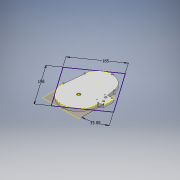
# Autodesk Inventor part: case part 1
Saved by Autodesk Inventor 2017 (Build 210142000, 142)
## iProperties
Created: 2018-04-16
Part Number: case part 1
Material: Generic
Document SubType Name: Modeling
Designer: RKL
Density: 1 g/cm^3
Appearance: Default
Mass: 277.252 g
Surface Area: 608.799 cm^2
Volume: 277.252 cm^3
Author: RKL
Autodesk Inventor part; units mm, degrees
(part 1 of 2)
ref_plane "YZ Plane" through (0, 0, 0) normal (1, 0, 0) x (0, 1, 0)
ref_plane "XZ Plane" through (0, 0, 0) normal (0, 1, 0) x (-1, 0, 0)
ref_plane "Work Plane1" through (0, 0, 0) normal (0, 0, 1) x (1, 0, 0)
sketch "Sketch1" plane through (0, 0, 0) normal (0, 0, 1) x (1, 0, 0)
  circle A0 centre (0, 0) radius 17.5 projected
  circle A1 centre (-1.6604, 79.9828) radius 17.5 projected
  circle A2 centre (0, 0) radius 6.7352 construction
  arc A3 (27.338, 58.5707) -> (27.6561, 62.122) centre (7.1943, 62.1651) ccw construction
  arc A4 (27.6561, 62.122) -> (26.5429, 62.6057) centre (0, 0) ccw construction
  arc A5 (26.5429, 62.6057) -> (24.1639, 59.95) centre (40.5363, 47.6767) ccw construction
  arc A6 (24.1639, 59.95) -> (23.09, 60.3717) centre (0, 0) ccw construction
  arc A7 (23.09, 60.3717) -> (23.1539, 63.9367) centre (2.7411, 62.5199) ccw construction
  arc A8 (23.1539, 63.9367) -> (22.009, 64.3397) centre (0, 0) ccw construction
  arc A9 (22.009, 64.3397) -> (19.8255, 61.5211) centre (37.0318, 50.447) ccw construction
  arc A10 (19.8255, 61.5211) -> (18.7243, 61.8651) centre (0, 0) ccw construction
  arc A11 (18.7243, 61.8651) -> (18.5338, 65.4255) centre (-1.726, 62.5562) ccw construction
  arc A12 (18.5338, 65.4255) -> (17.363, 65.7459) centre (0, 0) ccw construction
  arc A13 (17.363, 65.7459) -> (15.3861, 62.7787) centre (33.3386, 52.9603) ccw construction
  arc A14 (15.3861, 62.7787) -> (14.2631, 63.0433) centre (0, 0) ccw construction
  arc A15 (14.2631, 63.0433) -> (13.8191, 66.581) centre (-6.1843, 62.2737) ccw construction
  arc A16 (13.8191, 66.581) -> (12.6285, 66.8171) centre (0, 0) ccw construction
  arc A17 (12.6285, 66.8171) -> (10.8684, 63.7163) centre (29.4755, 55.2037) ccw construction
  arc A18 (10.8684, 63.7163) -> (9.7293, 63.9002) centre (0, 0) ccw construction
  arc A19 (9.7293, 63.9002) -> (9.0341, 67.3972) centre (-10.6111, 61.6738) ccw construction
  arc A20 (9.0341, 67.3972) -> (7.8297, 67.5477) centre (0, 0) ccw construction
  arc A21 (7.8297, 67.5477) -> (6.2952, 64.3293) centre (25.4622, 57.1658) ccw construction
  arc A22 (6.2952, 64.3293) -> (5.146, 64.4314) centre (0, 0) ccw construction
  arc A23 (5.146, 64.4314) -> (4.203, 67.87) centre (-14.9838, 60.7597) ccw construction
  arc A24 (4.203, 67.87) -> (2.9909, 67.9342) centre (0, 0) ccw construction
  arc A25 (2.9909, 67.9342) -> (1.6899, 64.6145) centre (21.3191, 58.8366) ccw construction
  arc A26 (1.6899, 64.6145) -> (0.5364, 64.6344) centre (0, 0) ccw construction
  arc A27 (0.5364, 64.6344) -> (-0.6495, 67.9969) centre (-19.2802, 59.536) ccw construction
  arc A28 (-0.6495, 67.9969) -> (-1.8631, 67.9745) centre (0, 0) ccw construction
  arc A29 (-1.8631, 67.9745) -> (-2.9239, 64.5704) centre (17.0675, 60.2076) ccw construction
  arc A30 (-2.9239, 64.5704) -> (-4.076, 64.508) centre (0, 0) ccw construction
  arc A31 (-4.076, 64.508) -> (-5.4987, 67.7773) centre (-23.4783, 58.0088) ccw construction
  arc A32 (-5.4987, 67.7773) -> (-6.7076, 67.6684) centre (0, 0) ccw construction
  arc A33 (-6.7076, 67.6684) -> (-7.5229, 64.1973) centre (12.7288, 61.2718) ccw construction
  arc A34 (-7.5229, 64.1973) -> (-8.6675, 64.0528) centre (0, 0) ccw construction
  arc A35 (-8.6675, 64.0528) -> (-10.3199, 67.2124) centre (-27.5568, 56.1861) ccw construction
  arc A36 (-10.3199, 67.2124) -> (-11.5179, 67.0174) centre (0, 0) ccw construction
  arc A37 (-11.5179, 67.0174) -> (-12.0835, 63.4971) centre (8.3253, 62.0238) ccw construction
  arc A38 (-12.0835, 63.4971) -> (-13.2149, 63.2713) centre (0, 0) ccw construction
  arc A39 (-13.2149, 63.2713) -> (-15.0884, 66.3049) centre (-31.4948, 54.0771) ccw construction
  arc A40 (-15.0884, 66.3049) -> (-16.2695, 66.025) centre (0, 0) ccw construction
  arc A41 (-16.2695, 66.025) -> (-16.5825, 62.4733) centre (3.8794, 62.4596) ccw construction
  arc A42 (-16.5825, 62.4733) -> (-17.695, 62.1674) centre (0, 0) ccw construction
  arc A43 (-17.695, 62.1674) -> (-19.7801, 65.0596) centre (-35.2724, 51.6925) ccw construction
  arc A44 (-19.7801, 65.0596) -> (-20.9382, 64.6961) centre (0, 0) ccw construction
  arc A45 (-20.9382, 64.6961) -> (-20.9971, 61.1311) centre (-0.5863, 62.5773) ccw construction
  arc A46 (-20.9971, 61.1311) -> (-22.0848, 60.7466) centre (0, 0) ccw construction
  arc A47 (-22.0848, 60.7466) -> (-24.371, 63.4827) centre (-38.8702, 49.0445) ccw construction
  arc A48 (-24.371, 63.4827) -> (-25.5002, 63.0376) centre (0, 0) ccw construction
  arc A49 (-25.5002, 63.0376) -> (-25.3046, 59.4775) centre (-5.049, 62.376) ccw construction
  arc A50 (-25.3046, 59.4775) -> (-26.3622, 59.0163) centre (0, 0) ccw construction
  arc A51 (-26.3622, 59.0163) -> (-28.8377, 61.5823) centre (-42.27, 46.1465) ccw construction
  arc A52 (-28.8377, 61.5823) -> (-29.9323, 61.0578) centre (0, 0) ccw construction
  arc A53 (-29.9323, 61.0578) -> (-29.4832, 57.5207) centre (-9.486, 61.8569) ccw construction
  arc A54 (-29.4832, 57.5207) -> (-30.5052, 56.9853) centre (0, 0) ccw construction
  arc A55 (-30.5052, 56.9853) -> (-33.1575, 59.3682) centre (-45.4544, 43.0135) ccw construction
  arc A56 (-33.1575, 59.3682) -> (-34.2119, 58.7669) centre (0, 0) ccw construction
  arc A57 (-34.2119, 58.7669) -> (-33.5116, 55.2708) centre (-13.8747, 61.0225) ccw construction
  arc A58 (-33.5116, 55.2708) -> (-34.4928, 54.6639) centre (0, 0) ccw construction
  arc A59 (-34.4928, 54.6639) -> (-37.3083, 56.8515) centre (-48.4071, 39.6612) ccw construction
  arc A60 (-37.3083, 56.8515) -> (-38.3171, 56.1765) centre (0, 0) ccw construction
  arc A61 (-38.3171, 56.1765) -> (-37.3692, 52.7393) centre (-18.1926, 59.8772) ccw construction
  arc A62 (-37.3692, 52.7393) -> (-38.3046, 52.0639) centre (0, 0) ccw construction
  arc A63 (-38.3046, 52.0639) -> (-41.269, 54.0451) centre (-51.1131, 36.1068) ccw construction
  arc A64 (-41.269, 54.0451) -> (-42.227, 53.2999) centre (0, 0) ccw construction
  arc A65 (-42.227, 53.2999) -> (-41.0363, 49.9391) centre (-22.4179, 58.4268) ccw construction
  arc A66 (-41.0363, 49.9391) -> (-41.9212, 49.1987) centre (0, 0) ccw construction
  arc A67 (-41.9212, 49.1987) -> (-45.0194, 50.9633) centre (-53.5587, 32.3685) ccw construction
  arc A68 (-45.0194, 50.9633) -> (-45.9218, 50.1516) centre (0, 0) ccw construction
  arc A69 (-45.9218, 50.1516) -> (-44.4944, 46.8843) centre (-26.5289, 56.6787) ccw construction
  arc A70 (-44.4944, 46.8843) -> (-45.3241, 46.0827) centre (0, 0) ccw construction
  arc A71 (-45.3241, 46.0827) -> (-48.5403, 47.6218) centre (-55.7314, 28.4651) ccw construction
  arc A72 (-48.5403, 47.6218) -> (-49.3826, 46.7478) centre (0, 0) ccw construction
  arc A73 (-49.3826, 46.7478) -> (-47.7257, 43.5907) centre (-30.5047, 54.6417) ccw construction
  arc A74 (-47.7257, 43.5907) -> (-48.4962, 42.7319) centre (0, 0) ccw construction
  arc A75 (-48.4962, 42.7319) -> (-51.814, 44.0376) centre (-57.6201, 24.4168) ccw construction
  arc A76 (-51.814, 44.0376) -> (-52.5917, 43.1058) centre (0, 0) ccw construction
  arc A77 (-52.5917, 43.1058) -> (-50.7138, 40.0749) centre (-34.3251, 52.3263) ccw construction
  arc A78 (-50.7138, 40.0749) -> (-51.4211, 39.1633) centre (0, 0) ccw construction
  arc A79 (-51.4211, 39.1633) -> (-54.8236, 40.2291) centre (-59.2152, 20.244) ccw construction
  arc A80 (-54.8236, 40.2291) -> (-55.5329, 39.2441) centre (0, 0) ccw construction
  arc A81 (-55.5329, 39.2441) -> (-53.4435, 36.3549) centre (-37.9705, 49.7443) ccw construction
  arc A82 (-53.4435, 36.3549) -> (-54.0839, 35.3952) centre (0, 0) ccw construction
  arc A83 (-54.0839, 35.3952) -> (-57.5538, 36.2155) centre (-60.5085, 15.9681) ccw construction
  arc A84 (-57.5538, 36.2155) -> (-58.191, 35.1825) centre (0, 0) ccw construction
  arc A85 (-58.191, 35.1825) -> (-55.9009, 32.4497) centre (-41.4225, 46.9088) ccw construction
  arc A86 (-55.9009, 32.4497) -> (-56.4712, 31.4467) centre (0, 0) ccw construction
  arc A87 (-56.4712, 31.4467) -> (-59.9907, 32.0174) centre (-61.4935, 11.6108) ccw construction
  arc A88 (-59.9907, 32.0174) -> (-60.5526, 30.9415) centre (0, 0) ccw construction
  arc A89 (-60.5526, 30.9415) -> (-58.0734, 28.3791) centre (-44.6634, 43.8342) ccw construction
  arc A90 (-58.0734, 28.3791) -> (-58.5707, 27.338) centre (0, 0) ccw construction
  arc A91 (-58.5707, 27.338) -> (-62.122, 27.6561) centre (-62.1651, 7.1943) ccw construction
  arc A92 (-62.122, 27.6561) -> (-62.6057, 26.5429) centre (0, 0) ccw construction
  arc A93 (-62.6057, 26.5429) -> (-59.95, 24.1639) centre (-47.6767, 40.5363) ccw construction
  arc A94 (-59.95, 24.1639) -> (-60.3717, 23.09) centre (0, 0) ccw construction
  arc A95 (-60.3717, 23.09) -> (-63.9367, 23.1539) centre (-62.5199, 2.7411) ccw construction
  arc A96 (-63.9367, 23.1539) -> (-64.3397, 22.009) centre (0, 0) ccw construction
  arc A97 (-64.3397, 22.009) -> (-61.5211, 19.8255) centre (-50.447, 37.0318) ccw construction
  arc A98 (-61.5211, 19.8255) -> (-61.8651, 18.7243) centre (0, 0) ccw construction
  arc A99 (-61.8651, 18.7243) -> (-65.4255, 18.5338) centre (-62.5562, -1.726) ccw construction
  arc A100 (-65.4255, 18.5338) -> (-65.7459, 17.363) centre (0, 0) ccw construction
  arc A101 (-65.7459, 17.363) -> (-62.7787, 15.3861) centre (-52.9603, 33.3386) ccw construction
  arc A102 (-62.7787, 15.3861) -> (-63.0433, 14.2631) centre (0, 0) ccw construction
  arc A103 (-63.0433, 14.2631) -> (-66.581, 13.8191) centre (-62.2737, -6.1843) ccw construction
  arc A104 (-66.581, 13.8191) -> (-66.8171, 12.6285) centre (0, 0) ccw construction
  arc A105 (-66.8171, 12.6285) -> (-63.7163, 10.8684) centre (-55.2037, 29.4755) ccw construction
  arc A106 (-63.7163, 10.8684) -> (-63.9002, 9.7293) centre (0, 0) ccw construction
  arc A107 (-63.9002, 9.7293) -> (-67.3972, 9.0341) centre (-61.6738, -10.6111) ccw construction
  arc A108 (-67.3972, 9.0341) -> (-67.5477, 7.8297) centre (0, 0) ccw construction
  arc A109 (-67.5477, 7.8297) -> (-64.3293, 6.2952) centre (-57.1658, 25.4622) ccw construction
  arc A110 (-64.3293, 6.2952) -> (-64.4314, 5.146) centre (0, 0) ccw construction
  arc A111 (-64.4314, 5.146) -> (-67.87, 4.203) centre (-60.7597, -14.9838) ccw construction
  arc A112 (-67.87, 4.203) -> (-67.9342, 2.9909) centre (0, 0) ccw construction
  arc A113 (-67.9342, 2.9909) -> (-64.6145, 1.6899) centre (-58.8366, 21.3191) ccw construction
  arc A114 (-64.6145, 1.6899) -> (-64.6344, 0.5364) centre (0, 0) ccw construction
  arc A115 (-64.6344, 0.5364) -> (-67.9969, -0.6495) centre (-59.536, -19.2802) ccw construction
  arc A116 (-67.9969, -0.6495) -> (-67.9745, -1.8631) centre (0, 0) ccw construction
  arc A117 (-67.9745, -1.8631) -> (-64.5704, -2.9239) centre (-60.2076, 17.0675) ccw construction
  arc A118 (-64.5704, -2.9239) -> (-64.508, -4.076) centre (0, 0) ccw construction
  arc A119 (-64.508, -4.076) -> (-67.7773, -5.4987) centre (-58.0088, -23.4783) ccw construction
  arc A120 (-67.7773, -5.4987) -> (-67.6684, -6.7076) centre (0, 0) ccw construction
  arc A121 (-67.6684, -6.7076) -> (-64.1973, -7.5229) centre (-61.2718, 12.7288) ccw construction
  arc A122 (-64.1973, -7.5229) -> (-64.0528, -8.6675) centre (0, 0) ccw construction
  arc A123 (-64.0528, -8.6675) -> (-67.2124, -10.3199) centre (-56.1861, -27.5568) ccw construction
  arc A124 (-67.2124, -10.3199) -> (-67.0174, -11.5179) centre (0, 0) ccw construction
  arc A125 (-67.0174, -11.5179) -> (-63.4971, -12.0835) centre (-62.0238, 8.3253) ccw construction
  arc A126 (-63.4971, -12.0835) -> (-63.2713, -13.2149) centre (0, 0) ccw construction
  arc A127 (-63.2713, -13.2149) -> (-66.3049, -15.0884) centre (-54.0771, -31.4948) ccw construction
  arc A128 (-66.3049, -15.0884) -> (-66.025, -16.2695) centre (0, 0) ccw construction
  arc A129 (-66.025, -16.2695) -> (-62.4733, -16.5825) centre (-62.4596, 3.8794) ccw construction
  arc A130 (-62.4733, -16.5825) -> (-62.1674, -17.695) centre (0, 0) ccw construction
  arc A131 (-62.1674, -17.695) -> (-65.0596, -19.7801) centre (-51.6925, -35.2724) ccw construction
  arc A132 (-65.0596, -19.7801) -> (-64.6961, -20.9382) centre (0, 0) ccw construction
  arc A133 (-64.6961, -20.9382) -> (-61.1311, -20.9971) centre (-62.5773, -0.5863) ccw construction
  arc A134 (-61.1311, -20.9971) -> (-60.7466, -22.0848) centre (0, 0) ccw construction
  arc A135 (-60.7466, -22.0848) -> (-63.4827, -24.371) centre (-49.0445, -38.8702) ccw construction
  arc A136 (-63.4827, -24.371) -> (-63.0376, -25.5002) centre (0, 0) ccw construction
  arc A137 (-63.0376, -25.5002) -> (-59.4775, -25.3046) centre (-62.376, -5.049) ccw construction
  arc A138 (-59.4775, -25.3046) -> (-59.0163, -26.3622) centre (0, 0) ccw construction
  arc A139 (-59.0163, -26.3622) -> (-61.5823, -28.8377) centre (-46.1465, -42.27) ccw construction
  arc A140 (-61.5823, -28.8377) -> (-61.0578, -29.9323) centre (0, 0) ccw construction
  arc A141 (-61.0578, -29.9323) -> (-57.5207, -29.4832) centre (-61.8569, -9.486) ccw construction
  arc A142 (-57.5207, -29.4832) -> (-56.9853, -30.5052) centre (0, 0) ccw construction
  arc A143 (-56.9853, -30.5052) -> (-59.3682, -33.1575) centre (-43.0135, -45.4544) ccw construction
  arc A144 (-59.3682, -33.1575) -> (-58.7669, -34.2119) centre (0, 0) ccw construction
  arc A145 (-58.7669, -34.2119) -> (-55.2708, -33.5116) centre (-61.0225, -13.8747) ccw construction
  arc A146 (-55.2708, -33.5116) -> (-54.6639, -34.4928) centre (0, 0) ccw construction
  arc A147 (-54.6639, -34.4928) -> (-56.8515, -37.3083) centre (-39.6612, -48.4071) ccw construction
  arc A148 (-56.8515, -37.3083) -> (-56.1765, -38.3171) centre (0, 0) ccw construction
  arc A149 (-56.1765, -38.3171) -> (-52.7393, -37.3692) centre (-59.8772, -18.1926) ccw construction
  arc A150 (-52.7393, -37.3692) -> (-52.0639, -38.3046) centre (0, 0) ccw construction
  arc A151 (-52.0639, -38.3046) -> (-54.0451, -41.269) centre (-36.1068, -51.1131) ccw construction
  arc A152 (-54.0451, -41.269) -> (-53.2999, -42.227) centre (0, 0) ccw construction
  arc A153 (-53.2999, -42.227) -> (-49.9391, -41.0363) centre (-58.4268, -22.4179) ccw construction
  arc A154 (-49.9391, -41.0363) -> (-49.1987, -41.9212) centre (0, 0) ccw construction
  arc A155 (-49.1987, -41.9212) -> (-50.9633, -45.0194) centre (-32.3685, -53.5587) ccw construction
  arc A156 (-50.9633, -45.0194) -> (-50.1516, -45.9218) centre (0, 0) ccw construction
  arc A157 (-50.1516, -45.9218) -> (-46.8843, -44.4944) centre (-56.6787, -26.5289) ccw construction
  arc A158 (-46.8843, -44.4944) -> (-46.0827, -45.3241) centre (0, 0) ccw construction
  arc A159 (-46.0827, -45.3241) -> (-47.6218, -48.5403) centre (-28.4651, -55.7314) ccw construction
  arc A160 (-47.6218, -48.5403) -> (-46.7478, -49.3826) centre (0, 0) ccw construction
  arc A161 (-46.7478, -49.3826) -> (-43.5907, -47.7257) centre (-54.6417, -30.5047) ccw construction
  arc A162 (-43.5907, -47.7257) -> (-42.7319, -48.4962) centre (0, 0) ccw construction
  arc A163 (-42.7319, -48.4962) -> (-44.0376, -51.814) centre (-24.4168, -57.6201) ccw construction
  arc A164 (-44.0376, -51.814) -> (-43.1058, -52.5917) centre (0, 0) ccw construction
  arc A165 (-43.1058, -52.5917) -> (-40.0749, -50.7138) centre (-52.3263, -34.3251) ccw construction
  arc A166 (-40.0749, -50.7138) -> (-39.1633, -51.4211) centre (0, 0) ccw construction
  arc A167 (-39.1633, -51.4211) -> (-40.2291, -54.8236) centre (-20.244, -59.2152) ccw construction
  arc A168 (-40.2291, -54.8236) -> (-39.2441, -55.5329) centre (0, 0) ccw construction
  arc A169 (-39.2441, -55.5329) -> (-36.3549, -53.4435) centre (-49.7443, -37.9705) ccw construction
  arc A170 (-36.3549, -53.4435) -> (-35.3952, -54.0839) centre (0, 0) ccw construction
  arc A171 (-35.3952, -54.0839) -> (-36.2155, -57.5538) centre (-15.9681, -60.5085) ccw construction
  arc A172 (-36.2155, -57.5538) -> (-35.1825, -58.191) centre (0, 0) ccw construction
  arc A173 (-35.1825, -58.191) -> (-32.4497, -55.9009) centre (-46.9088, -41.4225) ccw construction
  arc A174 (-32.4497, -55.9009) -> (-31.4467, -56.4712) centre (0, 0) ccw construction
  arc A175 (-31.4467, -56.4712) -> (-32.0174, -59.9907) centre (-11.6108, -61.4935) ccw construction
  arc A176 (-32.0174, -59.9907) -> (-30.9415, -60.5526) centre (0, 0) ccw construction
  arc A177 (-30.9415, -60.5526) -> (-28.3791, -58.0734) centre (-43.8342, -44.6634) ccw construction
  arc A178 (-28.3791, -58.0734) -> (-27.338, -58.5707) centre (0, 0) ccw construction
  arc A179 (-27.338, -58.5707) -> (-27.6561, -62.122) centre (-7.1943, -62.1651) ccw construction
  arc A180 (-27.6561, -62.122) -> (-26.5429, -62.6057) centre (0, 0) ccw construction
  arc A181 (-26.5429, -62.6057) -> (-24.1639, -59.95) centre (-40.5363, -47.6767) ccw construction
  arc A182 (-24.1639, -59.95) -> (-23.09, -60.3717) centre (0, 0) ccw construction
  arc A183 (-23.09, -60.3717) -> (-23.1539, -63.9367) centre (-2.7411, -62.5199) ccw construction
  arc A184 (-23.1539, -63.9367) -> (-22.009, -64.3397) centre (0, 0) ccw construction
  arc A185 (-22.009, -64.3397) -> (-19.8255, -61.5211) centre (-37.0318, -50.447) ccw construction
  arc A186 (-19.8255, -61.5211) -> (-18.7243, -61.8651) centre (0, 0) ccw construction
  arc A187 (-18.7243, -61.8651) -> (-18.5338, -65.4255) centre (1.726, -62.5562) ccw construction
  arc A188 (-18.5338, -65.4255) -> (-17.363, -65.7459) centre (0, 0) ccw construction
  arc A189 (-17.363, -65.7459) -> (-15.3861, -62.7787) centre (-33.3386, -52.9603) ccw construction
  arc A190 (-15.3861, -62.7787) -> (-14.2631, -63.0433) centre (0, 0) ccw construction
  arc A191 (-14.2631, -63.0433) -> (-13.8191, -66.581) centre (6.1843, -62.2737) ccw construction
  arc A192 (-13.8191, -66.581) -> (-12.6285, -66.8171) centre (0, 0) ccw construction
  arc A193 (-12.6285, -66.8171) -> (-10.8684, -63.7163) centre (-29.4755, -55.2037) ccw construction
  arc A194 (-10.8684, -63.7163) -> (-9.7293, -63.9002) centre (0, 0) ccw construction
  arc A195 (-9.7293, -63.9002) -> (-9.0341, -67.3972) centre (10.6111, -61.6738) ccw construction
  arc A196 (-9.0341, -67.3972) -> (-7.8297, -67.5477) centre (0, 0) ccw construction
  arc A197 (-7.8297, -67.5477) -> (-6.2952, -64.3293) centre (-25.4622, -57.1658) ccw construction
  arc A198 (-6.2952, -64.3293) -> (-5.146, -64.4314) centre (0, 0) ccw construction
  arc A199 (-5.146, -64.4314) -> (-4.203, -67.87) centre (14.9838, -60.7597) ccw construction
  arc A200 (-4.203, -67.87) -> (-2.9909, -67.9342) centre (0, 0) ccw construction
  arc A201 (-2.9909, -67.9342) -> (-1.6899, -64.6145) centre (-21.3191, -58.8366) ccw construction
  arc A202 (-1.6899, -64.6145) -> (-0.5364, -64.6344) centre (0, 0) ccw construction
  arc A203 (-0.5364, -64.6344) -> (0.6495, -67.9969) centre (19.2802, -59.536) ccw construction
  arc A204 (0.6495, -67.9969) -> (1.8631, -67.9745) centre (0, 0) ccw construction
  arc A205 (1.8631, -67.9745) -> (2.9239, -64.5704) centre (-17.0675, -60.2076) ccw construction
  arc A206 (2.9239, -64.5704) -> (4.076, -64.508) centre (0, 0) ccw construction
  arc A207 (4.076, -64.508) -> (5.4987, -67.7773) centre (23.4783, -58.0088) ccw construction
  arc A208 (5.4987, -67.7773) -> (6.7076, -67.6684) centre (0, 0) ccw construction
  arc A209 (6.7076, -67.6684) -> (7.5229, -64.1973) centre (-12.7288, -61.2718) ccw construction
  arc A210 (7.5229, -64.1973) -> (8.6675, -64.0528) centre (0, 0) ccw construction
  arc A211 (8.6675, -64.0528) -> (10.3199, -67.2124) centre (27.5568, -56.1861) ccw construction
  arc A212 (10.3199, -67.2124) -> (11.5179, -67.0174) centre (0, 0) ccw construction
  arc A213 (11.5179, -67.0174) -> (12.0835, -63.4971) centre (-8.3253, -62.0238) ccw construction
  arc A214 (12.0835, -63.4971) -> (13.2149, -63.2713) centre (0, 0) ccw construction
  arc A215 (13.2149, -63.2713) -> (15.0884, -66.3049) centre (31.4948, -54.0771) ccw construction
  arc A216 (15.0884, -66.3049) -> (16.2695, -66.025) centre (0, 0) ccw construction
  arc A217 (16.2695, -66.025) -> (16.5825, -62.4733) centre (-3.8794, -62.4596) ccw construction
  arc A218 (16.5825, -62.4733) -> (17.695, -62.1674) centre (0, 0) ccw construction
  arc A219 (17.695, -62.1674) -> (19.7801, -65.0596) centre (35.2724, -51.6925) ccw construction
  arc A220 (19.7801, -65.0596) -> (20.9382, -64.6961) centre (0, 0) ccw construction
  arc A221 (20.9382, -64.6961) -> (20.9971, -61.1311) centre (0.5863, -62.5773) ccw construction
  arc A222 (20.9971, -61.1311) -> (22.0848, -60.7466) centre (0, 0) ccw construction
  arc A223 (22.0848, -60.7466) -> (24.371, -63.4827) centre (38.8702, -49.0445) ccw construction
  arc A224 (24.371, -63.4827) -> (25.5002, -63.0376) centre (0, 0) ccw construction
  arc A225 (25.5002, -63.0376) -> (25.3046, -59.4775) centre (5.049, -62.376) ccw construction
  arc A226 (25.3046, -59.4775) -> (26.3622, -59.0163) centre (0, 0) ccw construction
  arc A227 (26.3622, -59.0163) -> (28.8377, -61.5823) centre (42.27, -46.1465) ccw construction
  arc A228 (28.8377, -61.5823) -> (29.9323, -61.0578) centre (0, 0) ccw construction
  arc A229 (29.9323, -61.0578) -> (29.4832, -57.5207) centre (9.486, -61.8569) ccw construction
  arc A230 (29.4832, -57.5207) -> (30.5052, -56.9853) centre (0, 0) ccw construction
  arc A231 (30.5052, -56.9853) -> (33.1575, -59.3682) centre (45.4544, -43.0135) ccw construction
  arc A232 (33.1575, -59.3682) -> (34.2119, -58.7669) centre (0, 0) ccw construction
  arc A233 (34.2119, -58.7669) -> (33.5116, -55.2708) centre (13.8747, -61.0225) ccw construction
  arc A234 (33.5116, -55.2708) -> (34.4928, -54.6639) centre (0, 0) ccw construction
  arc A235 (34.4928, -54.6639) -> (37.3083, -56.8515) centre (48.4071, -39.6612) ccw construction
  arc A236 (37.3083, -56.8515) -> (38.3171, -56.1765) centre (0, 0) ccw construction
  arc A237 (38.3171, -56.1765) -> (37.3692, -52.7393) centre (18.1926, -59.8772) ccw construction
  arc A238 (37.3692, -52.7393) -> (38.3046, -52.0639) centre (0, 0) ccw construction
  arc A239 (38.3046, -52.0639) -> (41.269, -54.0451) centre (51.1131, -36.1068) ccw construction
  arc A240 (41.269, -54.0451) -> (42.227, -53.2999) centre (0, 0) ccw construction
  arc A241 (42.227, -53.2999) -> (41.0363, -49.9391) centre (22.4179, -58.4268) ccw construction
  arc A242 (41.0363, -49.9391) -> (41.9212, -49.1987) centre (0, 0) ccw construction
  arc A243 (41.9212, -49.1987) -> (45.0194, -50.9633) centre (53.5587, -32.3685) ccw construction
  arc A244 (45.0194, -50.9633) -> (45.9218, -50.1516) centre (0, 0) ccw construction
  arc A245 (45.9218, -50.1516) -> (44.4944, -46.8843) centre (26.5289, -56.6787) ccw construction
  arc A246 (44.4944, -46.8843) -> (45.3241, -46.0827) centre (0, 0) ccw construction
  arc A247 (45.3241, -46.0827) -> (48.5403, -47.6218) centre (55.7314, -28.4651) ccw construction
  arc A248 (48.5403, -47.6218) -> (49.3826, -46.7478) centre (0, 0) ccw construction
  arc A249 (49.3826, -46.7478) -> (47.7257, -43.5907) centre (30.5047, -54.6417) ccw construction
  arc A250 (47.7257, -43.5907) -> (48.4962, -42.7319) centre (0, 0) ccw construction
  arc A251 (48.4962, -42.7319) -> (51.814, -44.0376) centre (57.6201, -24.4168) ccw construction
  arc A252 (51.814, -44.0376) -> (52.5917, -43.1058) centre (0, 0) ccw construction
  arc A253 (52.5917, -43.1058) -> (50.7138, -40.0749) centre (34.3251, -52.3263) ccw construction
  arc A254 (50.7138, -40.0749) -> (51.4211, -39.1633) centre (0, 0) ccw construction
  arc A255 (51.4211, -39.1633) -> (54.8236, -40.2291) centre (59.2152, -20.244) ccw construction
  arc A256 (54.8236, -40.2291) -> (55.5329, -39.2441) centre (0, 0) ccw construction
  arc A257 (55.5329, -39.2441) -> (53.4435, -36.3549) centre (37.9705, -49.7443) ccw construction
  arc A258 (53.4435, -36.3549) -> (54.0839, -35.3952) centre (0, 0) ccw construction
  arc A259 (54.0839, -35.3952) -> (57.5538, -36.2155) centre (60.5085, -15.9681) ccw construction
  arc A260 (57.5538, -36.2155) -> (58.191, -35.1825) centre (0, 0) ccw construction
  arc A261 (58.191, -35.1825) -> (55.9009, -32.4497) centre (41.4225, -46.9088) ccw construction
  arc A262 (55.9009, -32.4497) -> (56.4712, -31.4467) centre (0, 0) ccw construction
  arc A263 (56.4712, -31.4467) -> (59.9907, -32.0174) centre (61.4935, -11.6108) ccw construction
  arc A264 (59.9907, -32.0174) -> (60.5526, -30.9415) centre (0, 0) ccw construction
  arc A265 (60.5526, -30.9415) -> (58.0734, -28.3791) centre (44.6634, -43.8342) ccw construction
  arc A266 (58.0734, -28.3791) -> (58.5707, -27.338) centre (0, 0) ccw construction
  arc A267 (58.5707, -27.338) -> (62.122, -27.6561) centre (62.1651, -7.1943) ccw construction
  arc A268 (62.122, -27.6561) -> (62.6057, -26.5429) centre (0, 0) ccw construction
  arc A269 (62.6057, -26.5429) -> (59.95, -24.1639) centre (47.6767, -40.5363) ccw construction
  arc A270 (59.95, -24.1639) -> (60.3717, -23.09) centre (0, 0) ccw construction
  arc A271 (60.3717, -23.09) -> (63.9367, -23.1539) centre (62.5199, -2.7411) ccw construction
  arc A272 (63.9367, -23.1539) -> (64.3397, -22.009) centre (0, 0) ccw construction
  arc A273 (64.3397, -22.009) -> (61.5211, -19.8255) centre (50.447, -37.0318) ccw construction
  arc A274 (61.5211, -19.8255) -> (61.8651, -18.7243) centre (0, 0) ccw construction
  arc A275 (61.8651, -18.7243) -> (65.4255, -18.5338) centre (62.5562, 1.726) ccw construction
  arc A276 (65.4255, -18.5338) -> (65.7459, -17.363) centre (0, 0) ccw construction
  arc A277 (65.7459, -17.363) -> (62.7787, -15.3861) centre (52.9603, -33.3386) ccw construction
  arc A278 (62.7787, -15.3861) -> (63.0433, -14.2631) centre (0, 0) ccw construction
  arc A279 (63.0433, -14.2631) -> (66.581, -13.8191) centre (62.2737, 6.1843) ccw construction
  arc A280 (66.581, -13.8191) -> (66.8171, -12.6285) centre (0, 0) ccw construction
  arc A281 (66.8171, -12.6285) -> (63.7163, -10.8684) centre (55.2037, -29.4755) ccw construction
  arc A282 (63.7163, -10.8684) -> (63.9002, -9.7293) centre (0, 0) ccw construction
  arc A283 (63.9002, -9.7293) -> (67.3972, -9.0341) centre (61.6738, 10.6111) ccw construction
  arc A284 (67.3972, -9.0341) -> (67.5477, -7.8297) centre (0, 0) ccw construction
  arc A285 (67.5477, -7.8297) -> (64.3293, -6.2952) centre (57.1658, -25.4622) ccw construction
  arc A286 (64.3293, -6.2952) -> (64.4314, -5.146) centre (0, 0) ccw construction
  arc A287 (64.4314, -5.146) -> (67.87, -4.203) centre (60.7597, 14.9838) ccw construction
  arc A288 (67.87, -4.203) -> (67.9342, -2.9909) centre (0, 0) ccw construction
  arc A289 (67.9342, -2.9909) -> (64.6145, -1.6899) centre (58.8366, -21.3191) ccw construction
  arc A290 (64.6145, -1.6899) -> (64.6344, -0.5364) centre (0, 0) ccw construction
  arc A291 (64.6344, -0.5364) -> (67.9969, 0.6495) centre (59.536, 19.2802) ccw construction
  arc A292 (67.9969, 0.6495) -> (67.9745, 1.8631) centre (0, 0) ccw construction
  arc A293 (67.9745, 1.8631) -> (64.5704, 2.9239) centre (60.2076, -17.0675) ccw construction
  arc A294 (64.5704, 2.9239) -> (64.508, 4.076) centre (0, 0) ccw construction
  arc A295 (64.508, 4.076) -> (67.7773, 5.4987) centre (58.0088, 23.4783) ccw construction
  arc A296 (67.7773, 5.4987) -> (67.6684, 6.7076) centre (0, 0) ccw construction
  arc A297 (67.6684, 6.7076) -> (64.1973, 7.5229) centre (61.2718, -12.7288) ccw construction
  arc A298 (64.1973, 7.5229) -> (64.0528, 8.6675) centre (0, 0) ccw construction
  arc A299 (64.0528, 8.6675) -> (67.2124, 10.3199) centre (56.1861, 27.5568) ccw construction
  arc A300 (67.2124, 10.3199) -> (67.0174, 11.5179) centre (0, 0) ccw construction
  arc A301 (67.0174, 11.5179) -> (63.4971, 12.0835) centre (62.0238, -8.3253) ccw construction
  arc A302 (63.4971, 12.0835) -> (63.2713, 13.2149) centre (0, 0) ccw construction
  arc A303 (63.2713, 13.2149) -> (66.3049, 15.0884) centre (54.0771, 31.4948) ccw construction
  arc A304 (66.3049, 15.0884) -> (66.025, 16.2695) centre (0, 0) ccw construction
  arc A305 (66.025, 16.2695) -> (62.4733, 16.5825) centre (62.4596, -3.8794) ccw construction
  arc A306 (62.4733, 16.5825) -> (62.1674, 17.695) centre (0, 0) ccw construction
  arc A307 (62.1674, 17.695) -> (65.0596, 19.7801) centre (51.6925, 35.2724) ccw construction
  arc A308 (65.0596, 19.7801) -> (64.6961, 20.9382) centre (0, 0) ccw construction
  arc A309 (64.6961, 20.9382) -> (61.1311, 20.9971) centre (62.5773, 0.5863) ccw construction
  arc A310 (61.1311, 20.9971) -> (60.7466, 22.0848) centre (0, 0) ccw construction
  arc A311 (60.7466, 22.0848) -> (63.4827, 24.371) centre (49.0445, 38.8702) ccw construction
  arc A312 (63.4827, 24.371) -> (63.0376, 25.5002) centre (0, 0) ccw construction
  arc A313 (63.0376, 25.5002) -> (59.4775, 25.3046) centre (62.376, 5.049) ccw construction
  arc A314 (59.4775, 25.3046) -> (59.0163, 26.3622) centre (0, 0) ccw construction
  arc A315 (59.0163, 26.3622) -> (61.5823, 28.8377) centre (46.1465, 42.27) ccw construction
  arc A316 (61.5823, 28.8377) -> (61.0578, 29.9323) centre (0, 0) ccw construction
  arc A317 (61.0578, 29.9323) -> (57.5207, 29.4832) centre (61.8569, 9.486) ccw construction
  arc A318 (57.5207, 29.4832) -> (56.9853, 30.5052) centre (0, 0) ccw construction
  arc A319 (56.9853, 30.5052) -> (59.3682, 33.1575) centre (43.0135, 45.4544) ccw construction
  arc A320 (59.3682, 33.1575) -> (58.7669, 34.2119) centre (0, 0) ccw construction
  arc A321 (58.7669, 34.2119) -> (55.2708, 33.5116) centre (61.0225, 13.8747) ccw construction
  arc A322 (55.2708, 33.5116) -> (54.6639, 34.4928) centre (0, 0) ccw construction
  arc A323 (54.6639, 34.4928) -> (56.8515, 37.3083) centre (39.6612, 48.4071) ccw construction
  arc A324 (56.8515, 37.3083) -> (56.1765, 38.3171) centre (0, 0) ccw construction
  arc A325 (56.1765, 38.3171) -> (52.7393, 37.3692) centre (59.8772, 18.1926) ccw construction
  arc A326 (52.7393, 37.3692) -> (52.0639, 38.3046) centre (0, 0) ccw construction
  arc A327 (52.0639, 38.3046) -> (54.0451, 41.269) centre (36.1068, 51.1131) ccw construction
  arc A328 (54.0451, 41.269) -> (53.2999, 42.227) centre (0, 0) ccw construction
  arc A329 (53.2999, 42.227) -> (49.9391, 41.0363) centre (58.4268, 22.4179) ccw construction
  arc A330 (49.9391, 41.0363) -> (49.1987, 41.9212) centre (0, 0) ccw construction
  arc A331 (49.1987, 41.9212) -> (50.9633, 45.0194) centre (32.3685, 53.5587) ccw construction
  arc A332 (50.9633, 45.0194) -> (50.1516, 45.9218) centre (0, 0) ccw construction
  arc A333 (50.1516, 45.9218) -> (46.8843, 44.4944) centre (56.6787, 26.5289) ccw construction
  arc A334 (46.8843, 44.4944) -> (46.0827, 45.3241) centre (0, 0) ccw construction
  arc A335 (46.0827, 45.3241) -> (47.6218, 48.5403) centre (28.4651, 55.7314) ccw construction
  arc A336 (47.6218, 48.5403) -> (46.7478, 49.3826) centre (0, 0) ccw construction
  arc A337 (46.7478, 49.3826) -> (43.5907, 47.7257) centre (54.6417, 30.5047) ccw construction
  arc A338 (43.5907, 47.7257) -> (42.7319, 48.4962) centre (0, 0) ccw construction
  arc A339 (42.7319, 48.4962) -> (44.0376, 51.814) centre (24.4168, 57.6201) ccw construction
  arc A340 (44.0376, 51.814) -> (43.1058, 52.5917) centre (0, 0) ccw construction
  arc A341 (43.1058, 52.5917) -> (40.0749, 50.7138) centre (52.3263, 34.3251) ccw construction
  arc A342 (40.0749, 50.7138) -> (39.1633, 51.4211) centre (0, 0) ccw construction
  arc A343 (39.1633, 51.4211) -> (40.2291, 54.8236) centre (20.244, 59.2152) ccw construction
  arc A344 (40.2291, 54.8236) -> (39.2441, 55.5329) centre (0, 0) ccw construction
  arc A345 (39.2441, 55.5329) -> (36.3549, 53.4435) centre (49.7443, 37.9705) ccw construction
  arc A346 (36.3549, 53.4435) -> (35.3952, 54.0839) centre (0, 0) ccw construction
  arc A347 (35.3952, 54.0839) -> (36.2155, 57.5538) centre (15.9681, 60.5085) ccw construction
  arc A348 (36.2155, 57.5538) -> (35.1825, 58.191) centre (0, 0) ccw construction
  arc A349 (35.1825, 58.191) -> (32.4497, 55.9009) centre (46.9088, 41.4225) ccw construction
  arc A350 (32.4497, 55.9009) -> (31.4467, 56.4712) centre (0, 0) ccw construction
  arc A351 (31.4467, 56.4712) -> (32.0174, 59.9907) centre (11.6108, 61.4935) ccw construction
  arc A352 (32.0174, 59.9907) -> (30.9415, 60.5526) centre (0, 0) ccw construction
  arc A353 (30.9415, 60.5526) -> (28.3791, 58.0734) centre (43.8342, 44.6634) ccw construction
  arc A354 (28.3791, 58.0734) -> (27.338, 58.5707) centre (0, 0) ccw construction
  line L0 (-2.3049, 86.687) -> (5.0439, 80.6273) construction
  line L1 (5.0439, 80.6273) -> (-1.0158, 73.2785) construction
  line L2 (-1.0158, 73.2785) -> (-8.3646, 79.3382) construction
  line L3 (-8.3646, 79.3382) -> (-2.3049, 86.687) construction
  arc A355 (37.216, 46.5883) -> (38.5292, 48.1808) centre (-1.6604, 79.9828) ccw construction
  arc A356 (32.9073, 42.1458) -> (30.4447, 47.5651) centre (6.6438, 33.4802) ccw construction
  arc A357 (30.4447, 47.5651) -> (31.724, 48.8841) centre (-1.6604, 79.9828) ccw construction
  arc A358 (31.724, 48.8841) -> (37.216, 46.5883) centre (45.0744, 73.1046) ccw construction
  arc A359 (38.5292, 48.1808) -> (35.2291, 53.1349) centre (13.9958, 35.4145) ccw construction
  arc A360 (35.2291, 53.1349) -> (36.2802, 54.642) centre (-1.6604, 79.9828) ccw construction
  arc A361 (36.2802, 54.642) -> (42.0694, 53.257) centre (45.5725, 80.6905) ccw construction
  arc A362 (42.0694, 53.257) -> (43.1101, 55.0395) centre (-1.6604, 79.9828) ccw construction
  arc A363 (43.1101, 55.0395) -> (39.0581, 59.4) centre (20.9423, 38.503) ccw construction
  arc A364 (39.0581, 59.4) -> (39.8538, 61.0563) centre (-1.6604, 79.9828) ccw construction
  arc A365 (39.8538, 61.0563) -> (45.7903, 60.6178) centre (44.8473, 88.258) ccw construction
  arc A366 (45.7903, 60.6178) -> (46.5315, 62.5442) centre (-1.6604, 79.9828) ccw construction
  arc A367 (46.5315, 62.5442) -> (41.8325, 66.1983) centre (27.3034, 42.6659) ccw construction
  arc A368 (41.8325, 66.1983) -> (42.3523, 67.9607) centre (-1.6604, 79.9828) ccw construction
  arc A369 (42.3523, 67.9607) -> (48.2821, 68.4802) centre (42.9176, 95.6112) ccw construction
  arc A370 (48.2821, 68.4802) -> (48.7048, 70.5005) centre (-1.6604, 79.9828) ccw construction
  arc A371 (48.7048, 70.5005) -> (43.4805, 73.3535) centre (32.9144, 47.7953) ccw construction
  arc A372 (43.4805, 73.3535) -> (43.7108, 75.1765) centre (-1.6604, 79.9828) ccw construction
  arc A373 (43.7108, 75.1765) -> (49.4805, 76.6405) centre (39.8334, 102.5596) ccw construction
  arc A374 (49.4805, 76.6405) -> (49.5736, 78.7025) centre (-1.6604, 79.9828) ccw construction
  arc A375 (49.5736, 78.7025) -> (43.9593, 80.6805) centre (37.6299, 53.7583) ccw construction
  arc A376 (43.9593, 80.6805) -> (43.8942, 82.5168) centre (-1.6604, 79.9828) ccw construction
  arc A377 (43.8942, 82.5168) -> (49.3544, 84.8874) centre (35.6745, 108.9233) ccw construction
  arc A378 (49.3544, 84.8874) -> (49.1155, 86.9376) centre (-1.6604, 79.9828) ccw construction
  arc A379 (49.1155, 86.9376) -> (43.2566, 87.9893) centre (41.3278, 60.4005) ccw construction
  arc A380 (43.2566, 87.9893) -> (42.8978, 89.7915) centre (-1.6604, 79.9828) ccw construction
  arc A381 (42.8978, 89.7915) -> (47.907, 93.0072) centre (30.5486, 114.5375) ccw construction
  arc A382 (47.907, 93.0072) -> (47.3424, 94.9925) centre (-1.6604, 79.9828) ccw construction
  arc A383 (47.3424, 94.9925) -> (41.3906, 95.0908) centre (43.9123, 67.5498) ccw construction
  arc A384 (41.3906, 95.0908) -> (40.7474, 96.8121) centre (-1.6604, 79.9828) ccw construction
  arc A385 (40.7474, 96.8121) -> (45.1759, 100.7897) centre (24.5886, 119.2567) ccw construction
  arc A386 (45.1759, 100.7897) -> (44.3001, 102.6587) centre (-1.6604, 79.9828) ccw construction
  arc A387 (44.3001, 102.6587) -> (38.4096, 101.8011) centre (45.3165, 75.0212) ccw construction
  arc A388 (38.4096, 101.8011) -> (37.4986, 103.3968) centre (-1.6604, 79.9828) ccw construction
  arc A389 (37.4986, 103.3968) -> (41.2317, 108.0333) centre (17.9487, 122.9587) ccw construction
  arc A390 (41.2317, 108.0333) -> (40.0674, 109.7377) centre (-1.6604, 79.9828) ccw construction
  arc A391 (40.0674, 109.7377) -> (34.3908, 107.9462) centre (45.5041, 82.6211) ccw construction
  arc A392 (34.3908, 107.9462) -> (33.2356, 109.3752) centre (-1.6604, 79.9828) ccw construction
  arc A393 (33.2356, 109.3752) -> (36.1766, 114.5504) centre (10.8009, 125.5477) ccw construction
  arc A394 (36.1766, 114.5504) -> (34.754, 116.046) centre (-1.6604, 79.9828) ccw construction
  arc A395 (34.754, 116.046) -> (29.4383, 113.3671) centre (44.4701, 90.1526) ccw construction
  arc A396 (29.4383, 113.3671) -> (28.0688, 114.5922) centre (-1.6604, 79.9828) ccw construction
  arc A397 (28.0688, 114.5922) -> (30.1416, 120.1723) centre (3.3304, 126.9566) ccw construction
  arc A398 (30.1416, 120.1723) -> (28.4975, 121.4202) centre (-1.6604, 79.9828) ccw construction
  arc A399 (28.4975, 121.4202) -> (23.6804, 117.9234) centre (42.2414, 97.4208) ccw construction
  arc A400 (23.6804, 117.9234) -> (22.1321, 118.913) centre (-1.6604, 79.9828) ccw construction
  arc A401 (22.1321, 118.913) -> (23.2829, 124.7532) centre (-4.2694, 127.1489) ccw construction
  arc A402 (23.2829, 124.7532) -> (21.46, 125.7213) centre (-1.6604, 79.9828) ccw construction
  arc A403 (21.46, 125.7213) -> (17.2661, 121.497) centre (38.8756, 104.2373) ccw construction
  arc A404 (17.2661, 121.497) -> (15.5791, 122.2254) centre (-1.6604, 79.9828) ccw construction
  arc A405 (15.5791, 122.2254) -> (15.7782, 128.1747) centre (-11.8015, 126.1196) ccw construction
  arc A406 (15.7782, 128.1747) -> (13.8236, 128.8378) centre (-1.6604, 79.9828) ccw construction
  arc A407 (13.8236, 128.8378) -> (10.3617, 123.9954) centre (34.46, 110.4256) ccw construction
  arc A408 (10.3617, 123.9954) -> (8.5797, 124.4438) centre (-1.6604, 79.9828) ccw construction
  arc A409 (8.5797, 124.4438) -> (7.8219, 130.3479) centre (-19.0711, 123.8953) ccw construction
  arc A410 (7.8219, 130.3479) -> (5.7862, 130.6889) centre (-1.6604, 79.9828) ccw construction
  arc A411 (5.7862, 130.6889) -> (3.1459, 125.3539) centre (29.1088, 115.8255) ccw construction
  arc A412 (3.1459, 125.3539) -> (1.3151, 125.5106) centre (-1.6604, 79.9828) ccw construction
  arc A413 (1.3151, 125.5106) -> (-0.3801, 131.2168) centre (-25.8897, 120.5338) ccw construction
  arc A414 (-0.3801, 131.2168) -> (-2.4441, 131.2268) centre (-1.6604, 79.9828) ccw construction
  arc A415 (-2.4441, 131.2268) -> (-4.1944, 125.5373) centre (22.9608, 120.2971) ccw construction
  arc A416 (-4.1944, 125.5373) -> (-6.0267, 125.3984) centre (-1.6604, 79.9828) ccw construction
  arc A417 (-6.0267, 125.3984) -> (-8.6152, 130.7587) centre (-32.0808, 116.122) ccw construction
  arc A418 (-8.6152, 130.7587) -> (-10.6541, 130.4375) centre (-1.6604, 79.9828) ccw construction
  arc A419 (-10.6541, 130.4375) -> (-11.4691, 124.5409) centre (16.1751, 123.7245) ccw construction
  arc A420 (-11.4691, 124.5409) -> (-13.2553, 124.1098) centre (-1.6604, 79.9828) ccw construction
  arc A421 (-13.2553, 124.1098) -> (-16.6701, 128.9855) centre (-37.484, 110.7743) ccw construction
  arc A422 (-16.6701, 128.9855) -> (-18.6311, 128.3414) centre (-1.6604, 79.9828) ccw construction
  arc A423 (-18.6311, 128.3414) -> (-18.4897, 122.3905) centre (8.9275, 126.0191) ccw construction
  arc A424 (-18.4897, 122.3905) -> (-20.1836, 121.6784) centre (-1.6604, 79.9828) ccw construction
  arc A425 (-20.1836, 121.6784) -> (-24.3363, 125.9432) centre (-41.9594, 104.629) ccw construction
  arc A426 (-24.3363, 125.9432) -> (-26.1686, 124.9929) centre (-1.6604, 79.9828) ccw construction
  arc A427 (-26.1686, 124.9929) -> (-25.0744, 119.1417) centre (1.4056, 127.1214) ccw construction
  arc A428 (-25.0744, 119.1417) -> (-26.6322, 118.1672) centre (-1.6604, 79.9828) ccw construction
  arc A429 (-26.6322, 118.1672) -> (-31.4153, 121.7106) centre (-45.391, 97.8454) ccw construction
  arc A430 (-31.4153, 121.7106) -> (-33.0713, 120.4786) centre (-1.6604, 79.9828) ccw construction
  arc A431 (-33.0713, 120.4786) -> (-31.0528, 114.8787) centre (-6.1957, 127.0027) ccw construction
  arc A432 (-31.0528, 114.8787) -> (-32.434, 113.6669) centre (-1.6604, 79.9828) ccw construction
  arc A433 (-32.434, 113.6669) -> (-37.7236, 116.3972) centre (-47.6901, 90.5992) ccw construction
  arc A434 (-37.7236, 116.3972) -> (-39.1606, 114.9155) centre (-1.6604, 79.9828) ccw construction
  arc A435 (-39.1606, 114.9155) -> (-36.2698, 109.712) centre (-13.6795, 125.6663) ccw construction
  arc A436 (-36.2698, 109.712) -> (-37.4388, 108.2943) centre (-1.6604, 79.9828) ccw construction
  arc A437 (-37.4388, 108.2943) -> (-43.0978, 110.1407) centre (-48.797, 83.078) ccw construction
  arc A438 (-43.0978, 110.1407) -> (-44.2786, 108.4477) centre (-1.6604, 79.9828) ccw construction
  arc A439 (-44.2786, 108.4477) -> (-40.5906, 103.7752) centre (-20.852, 123.1467) ccw construction
  arc A440 (-40.5906, 103.7752) -> (-41.517, 102.1884) centre (-1.6604, 79.9828) ccw construction
  arc A441 (-41.517, 102.1884) -> (-47.3989, 103.1031) centre (-48.6832, 75.4767) ccw construction
  arc A442 (-47.3989, 103.1031) -> (-48.2928, 101.2426) centre (-1.6604, 79.9828) ccw construction
  arc A443 (-48.2928, 101.2426) -> (-43.903, 97.2223) centre (-27.5274, 119.5092) ccw construction
  arc A444 (-43.903, 97.2223) -> (-44.5629, 95.5074) centre (-1.6604, 79.9828) ccw construction
  arc A445 (-44.5629, 95.5074) -> (-50.5154, 95.4667) centre (-47.3514, 67.9921) ccw construction
  arc A446 (-50.5154, 95.4667) -> (-51.0992, 93.487) centre (-1.6604, 79.9828) ccw construction
  arc A447 (-51.0992, 93.487) -> (-46.1214, 90.2228) centre (-33.533, 114.848) ccw construction
  arc A448 (-46.1214, 90.2228) -> (-46.4976, 88.4243) centre (-1.6604, 79.9828) ccw construction
  arc A449 (-46.4976, 88.4243) -> (-52.3665, 87.4293) centre (-44.8363, 60.818) ccw construction
  arc A450 (-52.3665, 87.4293) -> (-52.6252, 85.3815) centre (-1.6604, 79.9828) ccw construction
  arc A451 (-64.6449, 6.7848) -> (64.3077, 9.4617) centre (0, 0) ccw
  arc A452 (52.7538, 87.9888) -> (-56.3599, 85.7237) centre (-1.6604, 79.9828) ccw
  line L4 (-64.6449, 6.7848) -> (-56.3599, 85.7237)
  line L5 (52.7538, 87.9888) -> (64.3077, 9.4617)
  arc A453 (57.7006, 88.7167) -> (-61.3326, 86.2456) centre (-1.6604, 79.9828) ccw
  line L6 (57.7006, 88.7167) -> (69.2544, 10.1895)
  arc A454 (-69.6176, 7.3067) -> (69.2544, 10.1895) centre (0, 0) ccw
  line L7 (-69.6176, 7.3067) -> (-61.3326, 86.2456)
  arc A455 (-52.9044, 79.1991) -> (-52.8313, 77.1363) centre (-1.6604, 79.9828) ccw projected
  arc A456 (-52.6252, 85.3815) -> (-47.1882, 82.9582) centre (-38.713, 109.2838) ccw projected
  arc A457 (-47.2711, 81.1226) -> (-52.9044, 79.1991) centre (-41.2029, 54.1403) ccw projected
  arc A458 (-52.8313, 77.1363) -> (-47.076, 75.6165) centre (-42.9334, 102.9607) ccw projected
  arc A459 (-46.8633, 73.7913) -> (-52.1151, 70.9891) centre (-36.5454, 48.1319) ccw projected
  arc A460 (-52.1151, 70.9891) -> (-51.712, 68.9648) centre (-1.6604, 79.9828) ccw projected
  arc A461 (-51.712, 68.9648) -> (-45.7874, 68.3878) centre (-46.0848, 96.0425) ccw projected
  arc A462 (-45.2848, 66.6204) -> (-50.019, 63.012) centre (-30.9844, 42.9484) ccw projected
  arc A463 (-50.019, 63.012) -> (-49.2964, 61.0786) centre (-1.6604, 79.9828) ccw projected
  arc A464 (-49.2964, 61.0786) -> (-43.356, 61.4595) centre (-48.0857, 88.7083) ccw projected
  arc A465 (-43.356, 61.4595) -> (-42.5764, 59.7956) centre (-1.6604, 79.9828) ccw projected
  arc A466 (-42.5764, 59.7956) -> (-46.6705, 55.4745) centre (-24.6639, 38.724) ccw projected
  arc A467 (-46.6705, 55.4745) -> (-45.6471, 53.682) centre (-1.6604, 79.9828) ccw projected
  arc A468 (-45.6471, 53.682) -> (-39.8448, 55.0109) centre (-48.8842, 81.1482) ccw projected
  arc A469 (-39.8448, 55.0109) -> (-38.8083, 53.4937) centre (-1.6604, 79.9828) ccw projected
  arc A470 (-38.8083, 53.4937) -> (-42.1562, 48.5718) centre (-17.7477, 35.5683) ccw projected
  arc A471 (-42.1562, 48.5718) -> (-40.8586, 46.9667) centre (-1.6604, 79.9828) ccw projected
  arc A472 (-40.8586, 46.9667) -> (-35.3445, 49.2091) centre (-48.4596, 73.5578) ccw projected
  arc A473 (-35.3445, 49.2091) -> (-34.0781, 47.8777) centre (-1.6604, 79.9828) ccw projected
  arc A474 (-34.0781, 47.8777) -> (-36.5931, 42.4826) centre (-10.4148, 33.5629) ccw projected
  arc A475 (-36.5931, 42.4826) -> (-35.0548, 41.1064) centre (-1.6604, 79.9828) ccw projected
  arc A476 (-35.0548, 41.1064) -> (-29.9719, 44.2043) centre (-46.8229, 66.1339) ccw projected
  arc A477 (-29.9719, 44.2043) -> (-28.5083, 43.0933) centre (-1.6604, 79.9828) ccw projected
  arc A478 (-28.5083, 43.0933) -> (-30.1253, 37.3646) centre (-2.8551, 32.7597) ccw projected
  arc A479 (-30.1253, 37.3646) -> (-28.3862, 36.253) centre (-1.6604, 79.9828) ccw projected
  arc A480 (-28.3862, 36.253) -> (-23.866, 40.1261) centre (-44.0166, 59.0687) ccw projected
  arc A481 (-23.866, 40.1261) -> (-22.2431, 39.2643) centre (-1.6604, 79.9828) ccw projected
  arc A482 (-22.2431, 39.2643) -> (-22.9202, 33.3504) centre (4.7354, 33.1796) ccw projected
  arc A483 (-22.9202, 33.3504) -> (-21.0253, 32.5321) centre (-1.6604, 79.9828) ccw projected
  arc A484 (-21.0253, 32.5321) -> (-17.185, 37.0802) centre (-40.1132, 52.5451) ccw projected
  arc A485 (-17.185, 37.0802) -> (-15.4449, 36.4899) centre (-1.6604, 79.9828) ccw projected
  arc A486 (-15.4449, 36.4899) -> (-15.1646, 30.5439) centre (12.1604, 34.8116) ccw projected
  arc A487 (-15.1646, 30.5439) -> (-13.1629, 30.0403) centre (-1.6604, 79.9828) ccw projected
  arc A488 (-13.1629, 30.0403) -> (-10.1019, 35.1455) centre (-35.2139, 46.7321) ccw projected
  arc A489 (-10.1019, 35.1455) -> (-8.2896, 34.8419) centre (-1.6604, 79.9828) ccw projected
  arc A490 (-8.2896, 34.8419) -> (-7.0592, 29.0179) centre (19.2274, 37.6136) ccw projected
  arc A491 (-7.0592, 29.0179) -> (-5.0026, 28.8419) centre (-1.6604, 79.9828) ccw projected
  arc A492 (-5.0026, 28.8419) -> (-2.8002, 34.372) centre (-29.4457, 41.7804) ccw projected
  arc A493 (-2.8002, 34.372) -> (-0.9627, 34.3631) centre (-1.6604, 79.9828) ccw projected
  arc A494 (-0.9627, 34.3631) -> (1.1861, 28.8119) centre (25.7534, 41.5129) ccw projected
  arc A495 (1.1861, 28.8119) -> (3.2442, 28.968) centre (-1.6604, 79.9828) ccw projected
  arc A496 (3.2442, 28.968) -> (4.5311, 34.7798) centre (-22.9578, 37.818) ccw projected
  arc A497 (4.5311, 34.7798) -> (6.3462, 35.0658) centre (-1.6604, 79.9828) ccw projected
  arc A498 (6.3462, 35.0658) -> (9.3576, 29.9311) centre (31.5694, 46.4085) ccw projected
  arc A499 (9.3576, 29.9311) -> (11.3641, 30.4154) centre (-1.6604, 79.9828) ccw projected
  arc A500 (11.3641, 30.4154) -> (11.702, 36.3584) centre (-15.9183, 34.9477) ccw projected
  arc A501 (11.702, 36.3584) -> (13.4477, 36.9318) centre (-1.6604, 79.9828) ccw projected
  arc A502 (13.4477, 36.9318) -> (17.2438, 32.3467) centre (36.5248, 52.1737) ccw projected
  arc A503 (17.2438, 32.3467) -> (19.1466, 33.1465) centre (-1.6604, 79.9828) ccw projected
  arc A504 (19.1466, 33.1465) -> (18.5268, 39.0668) centre (-8.5095, 33.2437) ccw projected
  arc A505 (18.5268, 39.0668) -> (20.1579, 39.9128) centre (-1.6604, 79.9828) ccw projected
  arc A506 (20.1579, 39.9128) -> (24.6404, 35.996) centre (40.4912, 58.6592) ccw projected
  arc A507 (24.6404, 35.996) -> (26.3902, 37.0907) centre (-1.6604, 79.9828) ccw projected
  arc A508 (26.3902, 37.0907) -> (24.8287, 42.8349) centre (-0.9233, 32.7503) ccw projected
  arc A509 (24.8287, 42.8349) -> (26.3031, 43.9316) centre (-1.6604, 79.9828) ccw projected
  arc A510 (26.3031, 43.9316) -> (31.3557, 40.7846) centre (43.3658, 65.6969) ccw projected
  arc A511 (31.3557, 40.7846) -> (32.9073, 42.1458) centre (-1.6604, 79.9828) ccw projected
  arc A512 (-47.1882, 82.9582) -> (-47.2711, 81.1226) centre (-1.6604, 79.9828) ccw projected
  arc A513 (-47.076, 75.6165) -> (-46.8633, 73.7913) centre (-1.6604, 79.9828) ccw projected
  arc A514 (-45.7874, 68.3878) -> (-45.2848, 66.6204) centre (-1.6604, 79.9828) ccw projected
  point P0 (-1.6604, 79.9828)
  dimension "d0" = 65
  dimension "d1" = 55
  dimension "d2" = 5
  constraints: 8 end point, 8 point on circle, 4 centre point, 4 tangent, 2 coincident, 3 other
  measures "d0" radius of A451
  measures "d1" radius of A452
  measures "d2" radial gap between concentric circles of A451 A454
extrude "Extrusion1" add sketch "Sketch1" along normal blind 10 contours L4 A452 L5 A451 | L6 A454 L7 A453
sketch "Sketch2" plane through (0, 0, 10) normal (0, 0, 1) x (1, 0, 0)
  circle A0 centre (-1.6604, 79.9828) radius 17.5 projected
  circle A1 centre (0, 0) radius 17.5 projected
  arc A2 (57.7006, 88.7167) -> (-61.3326, 86.2456) centre (-1.6604, 79.9828) ccw projected
  line L0 (-61.3326, 86.2456) -> (-69.6176, 7.3067) projected
  arc A3 (-69.6176, 7.3067) -> (69.2544, 10.1895) centre (0, 0) ccw projected
  line L1 (69.2544, 10.1895) -> (57.7006, 88.7167) projected
  circle A4 centre (-1.6604, 79.9828) radius 6.75
  circle A5 centre (0, 0) radius 6.75
  dimension "d5" = 13.5
  dimension "d44" = 13.5
  constraints: 2 centre point, 2 coincident
  measures "d5" diameter of A4
  measures "d44" diameter of A5
extrude "Extrusion2" add sketch "Sketch2" along normal blind 2 contours A0 | A1 | L1 A3 L0 A2 | A4